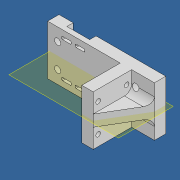
# Autodesk Inventor part: Linear_Unit_Mount
Saved by Autodesk Inventor 2020 (Build 240168000, 168)
## iProperties
Created: 2021-07-13
Part Number: Linear_Unit_Mount
Material: 一般
Document SubType Name: Modeling
Designer: ken113
Density: 1 g/cm^3
Appearance: 既定
Author: ken113
Autodesk Inventor part; units mm, degrees
ref_plane "YZ Plane" through (0, 0, 0) normal (1, 0, 0) x (0, 1, 0)
ref_plane "XZ Plane" through (0, 0, 0) normal (0, 1, 0) x (-1, 0, 0)
ref_plane "XY Plane" through (0, 0, 0) normal (0, 0, 1) x (1, 0, 0)
sketch "スケッチ1" plane through (0, 0, 0) normal (1, 0, 0) x (0, 1, 0)
  line L0 (-10, -10) -> (10, -10)
  line L1 (10, -10) -> (10, 10)
  line L2 (10, 10) -> (-10, 10)
  line L3 (-10, 10) -> (-10, -10)
  line L4 (-10, -10) -> (10, 10) construction
  line L5 (10, -10) -> (-10, 10) construction
  circle A0 centre (10, 10) radius 1.6
  circle A1 centre (-10, 10) radius 1.6
  circle A2 centre (-10, -10) radius 1.6
  circle A3 centre (10, -10) radius 1.6
  line L6 (-17.5, -15) -> (17.5, -15)
  line L7 (17.5, -15) -> (17.5, 15)
  line L8 (17.5, 15) -> (-17.5, 15)
  line L9 (-17.5, 15) -> (-17.5, -15)
  line L10 (-17.5, -15) -> (17.5, 15) construction
  line L11 (17.5, -15) -> (-17.5, 15) construction
  point P0 (0, 0)
  dimension "d0" = 20
  dimension "d1" = 20
  dimension "d2" = 3.2
  dimension "d3" = 3.2
  dimension "d4" = 3.2
  dimension "d5" = 3.2
  dimension "d6" = 15
  dimension "d7" = 35
  constraints: 24 end point, 4 centre point, 4 coincident, 4 midpoint, 4 parallel, 2 horizontal, 2 perpendicular
  measures "d0" distance of L2.end L1.end
  measures "d1" distance of L1.end L0.end
  measures "d2" diameter of A0
  measures "d3" diameter of A1
  measures "d4" diameter of A2
  measures "d5" diameter of A3
  measures "d6" distance from line of point (0, 0) L8
  measures "d7" distance of L6.start L6.end
extrude "押し出し1" add sketch "スケッチ1" along normal blind 8 contours A2 L3 A1 L2 A0 L1 A3 L0 | L9 L8 L7 L6
sketch "スケッチ2" plane through (8, 0, 0) normal (1, 0, 0) x (0, 0, -1)
  line L0 (-15, -17.5) -> (15, -17.5) projected
  line L1 (15, -17.5) -> (15, 17.5) projected
  line L2 (15, 17.5) -> (-15, 17.5) projected
  line L3 (-15, 17.5) -> (-15, -17.5) projected
  circle A0 centre (-10, 10) radius 1.6 projected
  circle A1 centre (-10, -10) radius 1.6 projected
  circle A2 centre (10, -10) radius 1.6 projected
  circle A3 centre (10, 10) radius 1.6 projected
  line L4 (15, -17.5) -> (15, 17.5) projected
  line L5 (15, -17.5) -> (21.5, -17.5)
  line L6 (21.5, -17.5) -> (21.5, 17.5)
  line L7 (21.5, 17.5) -> (15, 17.5)
  line L8 (15, 17.5) -> (15, -17.5)
  point P0 (0, 0)
  dimension "d10" = 21.5
  constraints: 8 end point, 2 parallel, 1 horizontal, 1 horizontal alignment, 1 perpendicular
  measures "d10" distance from line of L6 point (0, 0)
extrude "押し出し2" add sketch "スケッチ2" against normal up to surface (8 mm away) contours L1 L7 L6 L5
sketch "スケッチ3" plane through (8, 0, 0) normal (1, 0, 0) x (0, 0, -1)
  line L0 (-15, -17.5) -> (21.5, -17.5) projected
  line L1 (21.5, -17.5) -> (13.5, -17.5)
  line L2 (13.5, -17.5) -> (13.5, 17.5)
  line L3 (13.5, 17.5) -> (21.5, 17.5)
  line L4 (21.5, 17.5) -> (21.5, -17.5)
  point P0 (0, 0)
  point P1 (-15, 17.5)
  dimension "d13" = 8
  constraints: 8 end point, 2 parallel, 1 horizontal, 1 horizontal alignment, 1 perpendicular
  measures "d13" distance between parallel lines of L4 L2
extrude "押し出し3" add sketch "スケッチ3" along normal blind 80
sketch "スケッチ4" plane through (0, -17.5, 15) normal (0, -1, 0) x (1, 0, 0)
  line L0 (0, -3.4) -> (0, -6.6) projected
  line L1 (0, -23.4) -> (0, -26.6) projected
  line L2 (0, 0) -> (0, -36.5) projected
  line L3 (88, -36.5) -> (0, -36.5) projected
  line L4 (88, -28.5) -> (88, -36.5) projected
  line L5 (8, -28.5) -> (88, -28.5) projected
  line L6 (8, 0) -> (8, -28.5) projected
  line L7 (0, 0) -> (8, 0) projected
  line L8 (39, -36.5) -> (23, -36.5)
  line L9 (23, -36.5) -> (23, -32)
  line L10 (23, -32) -> (39, -32)
  line L11 (39, -32) -> (39, -36.5)
  point P0 (0, -15)
  dimension "d16" = 17
  dimension "d17" = 23
  dimension "d18" = 16
  constraints: 8 end point, 2 parallel, 1 horizontal, 1 perpendicular, 1 point on line
  measures "d16" distance from line of L10 point (0, -15)
  measures "d17" distance from line of L9 L1.start
  measures "d18" distance of L9.end L10.end
extrude "押し出し4" cut sketch "スケッチ4" against normal through all contours L9 L10 L11 L3
sketch "スケッチ5" plane through (39, -17.5, -17) normal (0, 0, -1) x (-1, 0, 0)
  line L0 (0, 0) -> (0, 35) projected
  line L1 (0, 35) -> (-49, 35) projected
  line L2 (-49, 0) -> (-49, 35) projected
  line L3 (-49, 0) -> (0, 0) projected
  line L4 (16, 35) -> (16, 0) projected
  line L5 (16, 0) -> (39, 0) projected
  line L6 (39, 35) -> (39, 0) projected
  line L7 (39, 35) -> (16, 35) projected
  line L8 (0, 35) -> (16, 35) projected
  line L9 (0, 0) -> (0, 35) projected
  line L10 (16, 0) -> (0, 0) projected
  line L11 (16, 0) -> (16, 35) projected
  line L12 (0, 0) -> (0, 35) projected
  line L13 (16, 35) -> (16, 0) projected
  line L14 (0, 10) -> (16, 10)
  line L15 (16, 10) -> (16, 25)
  line L16 (16, 25) -> (0, 25)
  line L17 (0, 25) -> (0, 10)
  point P0 (39, 17.5)
  point P1 (0, 25)
  point P2 (0, 10)
  point P3 (16, 10)
  dimension "d21" = 10
  dimension "d22" = 10
  constraints: 8 end point, 2 parallel, 2 point on line, 1 horizontal, 1 perpendicular
  measures "d21" distance between parallel lines of L14 L10
  measures "d22" distance between parallel lines of L8 L16
extrude "押し出し5" add sketch "スケッチ5" along normal up to surface (4.5 mm away) contours L0 L16 L4 L14
sketch "スケッチ6" plane through (39, -17.5, -17) normal (0, 0, -1) x (-1, 0, 0)
  line L0 (0, 25) -> (16, 25) projected
  line L1 (16, 25) -> (16, 35) projected
  line L2 (0, 35) -> (16, 35) projected
  line L3 (0, 25) -> (0, 35) projected
  line L4 (16, 10) -> (0, 10) projected
  line L5 (0, 0) -> (0, 10) projected
  line L6 (16, 0) -> (0, 0) projected
  line L7 (16, 0) -> (16, 10) projected
  line L8 (0, 0) -> (0, 10) projected
  line L9 (16, 10) -> (16, 0) projected
  line L10 (0, 4) -> (16, 4)
  line L11 (16, 4) -> (16, 6)
  line L12 (16, 6) -> (0, 6)
  line L13 (0, 6) -> (0, 4)
  line L14 (0, 25) -> (0, 35) projected
  line L15 (16, 35) -> (16, 25) projected
  line L16 (0, 29) -> (16, 29)
  line L17 (16, 29) -> (16, 31)
  line L18 (16, 31) -> (0, 31)
  line L19 (0, 31) -> (0, 29)
  line L20 (9.5, 4) -> (6.5, 4)
  line L21 (6.5, 4) -> (6.5, 31)
  line L22 (6.5, 31) -> (9.5, 31)
  line L23 (9.5, 31) -> (9.5, 4)
  point P0 (39, 17.5)
  point P1 (6.5, 29)
  point P2 (0, 31)
  point P3 (0, 29)
  point P4 (9.5, 31)
  point P5 (9.5, 29)
  point P6 (16, 29)
  point P7 (9.5, 6)
  point P8 (16, 4)
  point P9 (16, 6)
  point P10 (6.5, 4)
  point P11 (6.5, 6)
  point P12 (0, 6)
  point P13 (0, 4)
  dimension "d25" = 2
  dimension "d26" = 2
  dimension "d27" = 4
  dimension "d28" = 4
  dimension "d29" = 6.5
  dimension "d30" = 6.5
  constraints: 24 end point, 6 parallel, 6 point on line, 3 horizontal, 3 perpendicular
  measures "d25" distance between parallel lines of L12 L10
  measures "d26" distance between parallel lines of L18 L16
  measures "d27" distance between parallel lines of L10 L6
  measures "d28" distance between parallel lines of L2 L18
  measures "d29" distance between parallel lines of L23 L7
  measures "d30" distance between parallel lines of L5 L21
extrude "押し出し6" cut sketch "スケッチ6" against normal blind 8 contours L3 L18 L21 L16 | L23 L18 L1 L16 | L21 L10 L5 L12 | L12 L7 L10 L23
chamfer "面取り1" distance 4.5 angle 45 2 edges at (31, -7.5, -21.5) (31, 7.5, -21.5)
fillet "フィレット1" radius 0.5 16 edges at (39, -13.5, -15.25) (39, -11.5, -15.25) (32.5, -13.5, -15.25) (32.5, -11.5, -15.25) (29.5, -11.5, -15.25) (29.5, -13.5, -15.25) (23, -13.5, -15.25) (23, -11.5, -15.25) (23, 11.5, -15.25) (23, 13.5, -15.25) (29.5, 11.5, -15.25) (29.5, 13.5, -15.25) (32.5, 11.5, -15.25) (32.5, 13.5, -15.25) (39, 13.5, -15.25) (39, 11.5, -15.25)
chamfer "面取り2" distance 5 angle 45 1 edges at (0, 0, -21.5)
sketch "スケッチ7" plane through (88, -17.5, -21.5) normal (0, 0, -1) x (-1, 0, 0)
  line L0 (83, 35) -> (83, 0) projected
  line L1 (83, 35) -> (65, 35) projected
  line L2 (65, 35) -> (65, 20.5) projected
  line L3 (49, 20.5) -> (65, 20.5) projected
  line L4 (49, 20.5) -> (49, 35) projected
  line L5 (49, 35) -> (0, 35) projected
  line L6 (0, 0) -> (0, 35) projected
  line L7 (0, 0) -> (49, 0) projected
  line L8 (49, 0) -> (49, 14.5) projected
  line L9 (65, 14.5) -> (49, 14.5) projected
  line L10 (65, 14.5) -> (65, 0) projected
  line L11 (65, 0) -> (83, 0) projected
  line L12 (68, 9) -> (13, 9)
  line L13 (13, 9) -> (13, 26)
  line L14 (13, 26) -> (68, 26)
  line L15 (68, 26) -> (68, 9)
  line L16 (68, 9) -> (13, 26) construction
  line L17 (13, 9) -> (68, 26) construction
  line L18 (88, 0) -> (88, 35) projected
  point P0 (88, 17.5)
  point P1 (40.5, 17.5)
  dimension "d40" = 55
  dimension "d41" = 17
  dimension "d42" = 20
  constraints: 12 end point, 2 midpoint, 2 parallel, 1 horizontal, 1 perpendicular
  measures "d40" distance of L13.end L14.end
  measures "d41" distance of L12.end L13.end
  measures "d42" distance from line of L14.end L18
hole "穴1" at (75, -8.5, -21.5) at (75, 8.5, -21.5) at (20, -8.5, -21.5) at (20, 8.5, -21.5) direction (0, 0, 1) diameter 4.4 depth 8.8
sketch "スケッチ8" plane through (0, 17.5, 15) normal (0, 1, 0) x (1, 0, 0)
  line L0 (0, 0) -> (8, 0)
  line L1 (8, 0) -> (8, 39.6409)
  line L2 (8, 39.6409) -> (0, 39.6409)
  line L3 (0, 39.6409) -> (0, 0)
  point P0 (0, 15)
  dimension "d50" = 8
  constraints: 8 end point, 2 parallel, 1 horizontal, 1 perpendicular
  measures "d50" distance of L0.start L0.end
extrude "押し出し7" cut sketch "スケッチ8" against normal through all
sketch "スケッチ9" plane through (88, 17.5, -13.5) normal (0, 1, 0) x (1, 0, 0)
  line L0 (-80, 0) -> (0, 0) projected
  line L1 (-24, 0) -> (-16, 0)
  line L2 (-16, 0) -> (-16, -27)
  line L3 (-16, -27) -> (-24, -27)
  line L4 (-24, -27) -> (-24, 0)
  line L5 (0, 8) -> (0, 0) projected
  point P0 (-88, -13.5)
  point P1 (-16, 0)
  dimension "d53" = 24
  dimension "d54" = 8
  dimension "d55" = 27
  constraints: 8 end point, 2 parallel, 1 horizontal, 1 perpendicular, 1 point on line
  measures "d53" distance between parallel lines of L4 L5
  measures "d54" distance of L2.end L3.end
  measures "d55" distance of L3.end L1.start
extrude "押し出し8" add sketch "スケッチ9" against normal up to surface (35 mm away)
sketch "スケッチ10" plane through (72, 17.5, 13.5) normal (1, 0, 0) x (0, 0, -1)
  line L0 (23.5, -7.5) -> (3.5, -7.5)
  line L1 (3.5, -7.5) -> (3.5, -27.5)
  line L2 (3.5, -27.5) -> (23.5, -27.5)
  line L3 (23.5, -27.5) -> (23.5, -7.5)
  line L4 (23.5, -7.5) -> (3.5, -27.5) construction
  line L5 (3.5, -7.5) -> (23.5, -27.5) construction
  point P0 (13.5, -17.5)
  dimension "d58" = 20
  dimension "d59" = 20
  constraints: 12 end point, 2 midpoint, 2 parallel, 1 horizontal, 1 perpendicular
  measures "d58" distance of L2.end L1.end
  measures "d59" distance of L1.end L0.end
hole "穴2" at (72, -10, -10) at (72, 10, -10) at (72, 10, 10) at (72, -10, 10) direction (-1, 0, 0) diameter 3.3 depth 8.8
ref_plane "作業平面1" through (88, 0, -13.5) normal (0, 1, 0) x (1, 0, 0)
sketch "スケッチ11" plane through (88, 0, -13.5) normal (0, 1, 0) x (1, 0, 0)
  line L0 (-80, 8) -> (-80, 0) projected
  line L1 (-80, 0) -> (-24, 0) projected
  line L2 (-24, 0) -> (-24, -27) projected
  line L3 (-24, -27) -> (-16, -27) projected
  line L4 (-16, -27) -> (-16, 0) projected
  line L5 (-16, 0) -> (0, 0) projected
  line L6 (0, 8) -> (0, 0) projected
  line L7 (-49, 8) -> (0, 8) projected
  line L8 (-49, 8) -> (-49, 3.5) projected
  line L9 (-49, 3.5) -> (-65, 3.5) projected
  line L10 (-65, 3.5) -> (-65, 8) projected
  line L11 (-80, 8) -> (-65, 8) projected
  line L12 (-16, -27) -> (-16, 0) projected
  line L13 (0, 0) -> (-16, -27)
  point P0 (-88, -13.5)
  constraints: 2 end point
extrude "押し出し9" add sketch "スケッチ11" along normal mid plane 8 contours L4 L5 L13
fillet "フィレット2" radius 5 2 edges at (80, 4, -13.5) (80, -4, -13.5)
sketch "スケッチ12" plane through (88, 17.5, -13.5) normal (0, 1, 0) x (1, 0, 0)
  line L0 (-65, 8) -> (-80, 8) projected
  line L1 (-80, 8) -> (-75, 8)
  line L2 (-75, 8) -> (-75, -7.2695)
  line L3 (-75, -7.2695) -> (-80, -7.2695)
  line L4 (-80, -7.2695) -> (-80, 8)
  point P0 (-88, -13.5)
  dimension "d71" = 5
  constraints: 8 end point, 2 parallel, 1 horizontal, 1 perpendicular
  measures "d71" distance of L2.end L3.end
extrude "押し出し10" cut sketch "スケッチ12" against normal blind 80
